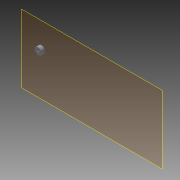
# Autodesk Inventor part: offsetWasher01
Saved by Autodesk Inventor 2013 (Build 170138000, 138)
## iProperties
Created: 2014-04-30
Part Number: offsetWasher01
Material: Wood (Birch)
Document SubType Name: Modeling
Designer: Nano
Mass: 0.414768 g
Surface Area: 5.54211 cm^2
Volume: 0.754123 cm^3
Density: 0.55 g/cm^3
Author: Nano
Autodesk Inventor part; units mm, degrees
ref_plane "YZ Plane" through (0, 0, 0) normal (1, 0, 0) x (0, 1, 0)
ref_plane "XZ Plane" through (0, 0, 0) normal (0, 1, 0) x (-1, 0, 0)
ref_plane "XY Plane" through (0, 0, 0) normal (0, 0, 1) x (1, 0, 0)
ref_plane "Work Plane1" through (0, 0, 0) normal (0, 0, 1) x (1, 0, 0)
sketch "Sketch1" plane through (0, 0, 0) normal (0, 0, 1) x (1, 0, 0)
  circle A0 centre (-93.6406, 22.5937) radius 1.5875 projected
  circle A1 centre (-93.6406, 22.5937) radius 6.35
  point P0 (0, 0)
  dimension "d0" = 12.7
  constraints: 1 centre point
  measures "d0" diameter of A1
extrude "Extrusion1" add sketch "Sketch1" along normal blind 6.35
body "Solid1"
